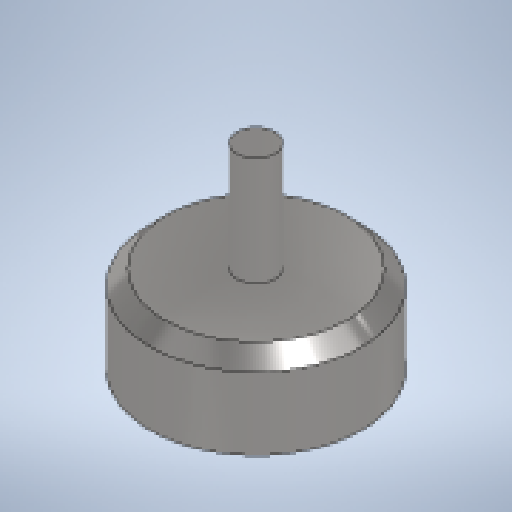
# Autodesk Inventor part: CAN
Saved by Autodesk Inventor 2023.2 (Build 272271000, 271)
## iProperties
Created: 2024-01-31
Part Number: CAN
Material: Stainless Steel
Document SubType Name: Modeling
Designer: Nathan Cai
Density: 8 g/cm^3
Appearance: Smooth - Black
Author: Nathan Cai
Autodesk Inventor part; units mm, degrees
ref_plane "YZ Plane" through (0, 0, 0) normal (1, 0, 0) x (0, 1, 0)
ref_plane "XZ Plane" through (0, 0, 0) normal (0, 1, 0) x (-1, 0, 0)
ref_plane "XY Plane" through (0, 0, 0) normal (0, 0, 1) x (1, 0, 0)
sketch "Sketch1" plane through (0, 0, 0) normal (0, 0, 1) x (1, 0, 0)
  line L0 (0, 0) -> (13.925, 0)
  line L1 (13.925, 0) -> (13.925, -11.5)
  line L2 (13.925, -11.5) -> (0, -11.5) construction
  line L3 (0, -11.5) -> (0, 0) construction
  line L4 (13.925, 0) -> (0, 0)
  line L5 (0, 0) -> (0, -3.5)
  line L6 (0, -3.5) -> (13.925, -3.5)
  line L7 (13.925, -3.5) -> (13.925, 0)
  line L8 (13.925, 0) -> (11.925, 0)
  line L9 (11.925, 0) -> (11.925, -6)
  line L10 (11.925, -6) -> (13.925, -6)
  line L11 (13.925, -6) -> (13.925, 0)
  line L12 (13.925, -6) -> (13.175, -6)
  line L13 (13.175, -6) -> (13.175, -11.5)
  line L14 (13.175, -11.5) -> (13.925, -11.5)
  line L15 (13.925, -11.5) -> (13.925, -6)
  line L16 (0, 0) -> (2.5, 0)
  line L17 (2.5, 0) -> (2.5, 14.25)
  line L18 (2.5, 14.25) -> (0, 14.25)
  line L19 (0, 14.25) -> (0, 0)
  line L20 (0, -3.5) -> (2, -3.5)
  line L21 (2, -3.5) -> (2, -6.5)
  line L22 (2, -6.5) -> (0, -6.5)
  line L23 (0, -6.5) -> (0, -3.5)
  line L24 (2, -6.5) -> (4.5, -3.5)
  line L25 (0, -3.5) -> (1.5, -3.5)
  line L26 (1.5, -3.5) -> (1.5, -6.5)
  line L27 (1.5, -6.5) -> (0, -6.5)
  line L28 (0, -6.5) -> (0, -3.5)
  line L29 (1.5, -6.5) -> (0, -6.5)
  line L30 (0, -6.5) -> (0, -0.5)
  line L31 (0, -0.5) -> (1.5, -0.5)
  line L32 (1.5, -0.5) -> (1.5, -6.5)
  point P0 (11.925, -3.5)
  point P1 (1.5, -3.5)
  point P2 (1.5, -3.5)
  dimension "d0" = 13.925
  dimension "d1" = 11.5
  dimension "d2" = 3.5
  dimension "d3" = 2
  dimension "d5" = 5.5
  dimension "d6" = 0.75
  dimension "d7" = 2.5
  dimension "d8" = 14.25
  dimension "d13" = 2
  dimension "d14" = 3
  dimension "d15" = 4.5
  dimension "d16" = 1.5
  dimension "d53" = 6
  constraints: 66 end point, 16 parallel, 8 horizontal, 8 perpendicular, 5 point on line
  measures "d0" distance of L1.end L2.end
  measures "d1" distance of L0.end L1.end
  measures "d2" distance of L5.end L4.end
  measures "d3" distance of L10.end L9.end
  measures "d5" distance between parallel lines of L2 L10
  measures "d6" distance of L14.end L13.end
  measures "d7" distance of L18.end L17.end
  measures "d8" distance of L17.end L16.end
  measures "d13" distance of L21.end L22.end
  measures "d14" distance of L20.end L21.end
  measures "d15" distance from line of L3 L24.end
  measures "d16" distance of L26.end L27.end
  measures "d53" distance of L29.end L30.end
revolve "Revolution1" add sketch "Sketch1" angle 360 about axis through (0, 14.25, 0) along (0, -1, 0) contours L19 L18 L17 L0 | L0 L9 L6 L32 L31 L5 | L0 L1 L6 L9 | L6 L1 L10 L9 | L6 L21 L22 L26 | L24 L21 L6 | L1 L14 L13 L10
chamfer "Chamfer1" distance 2 angle 45 1 edges at (-13.925, 0, 0)
sketch "Sketch4" plane through (0, -3.5, 0) normal (0, -1, 0) x (1, 0, 0)
  line L0 (0, 0) -> (0, 13.925) construction
  circle A0 centre (0, 0) radius 13.925 projected
  circle A1 centre (0, 0) radius 11.925 projected
  circle A2 centre (0, 0) radius 4.5 projected
  arc A3 (-1.9387, 6.0086) -> (1.9387, 6.0086) centre (0, 6.5) ccw
  line L1 (-1, -13.889) -> (1, -13.889) construction
  line L2 (1, -13.889) -> (1, -4.3875) construction
  line L3 (1, -4.3875) -> (-1, -4.3875) construction
  line L4 (-1, -4.3875) -> (-1, -13.889) construction
  line L5 (-1, -13.889) -> (1, -4.3875) construction
  line L6 (1, -13.889) -> (-1, -4.3875) construction
  circle A4 centre (0, 0) radius 4.5 projected
  circle A5 centre (0, 0) radius 11.925 projected
  line L7 (-3.319, 11.4538) -> (-1.9387, 6.0086)
  line L8 (3.4812, 12.0939) -> (1.9387, 6.0086)
  line L9 (2.0542, -4.0038) -> (8.1617, -11.2824) construction
  line L10 (9.6938, -9.9968) -> (3.5863, -2.7182) construction
  line L11 (4.1472, -1.7467) -> (13.5044, -3.3966) construction
  line L12 (13.8517, -1.427) -> (4.4945, 0.2229) construction
  line L13 (4.2997, 1.3277) -> (12.5283, 6.0785) construction
  line L14 (11.5283, 7.8105) -> (3.2997, 3.0598) construction
  line L15 (2.4403, 3.7809) -> (5.69, 12.7094) construction
  line L16 (3.8106, 13.3935) -> (0.5609, 4.4649) construction
  line L17 (-0.5609, 4.4649) -> (-3.8106, 13.3935) construction
  line L18 (-5.69, 12.7094) -> (-2.4403, 3.7809) construction
  line L19 (-3.2997, 3.0598) -> (-11.5283, 7.8105) construction
  line L20 (-12.5283, 6.0785) -> (-4.2997, 1.3277) construction
  line L21 (-4.4945, 0.2229) -> (-13.8517, -1.427) construction
  line L22 (-13.5044, -3.3966) -> (-4.1472, -1.7467) construction
  line L23 (-3.5863, -2.7182) -> (-9.6938, -9.9968) construction
  line L24 (-8.1617, -11.2824) -> (-2.0542, -4.0038) construction
  line L25 (-5.1071, 11.5022) -> (-2.3771, 5.849)
  arc A6 (-5.3474, 3.3567) -> (-2.3771, 5.849) centre (-4.1781, 4.9793) ccw
  line L26 (-9.9049, 6.6407) -> (-5.3474, 3.3567)
  line L27 (-11.3057, 5.5284) -> (-5.5806, 2.9526)
  arc A7 (-6.2539, -0.8659) -> (-5.5806, 2.9526) centre (-6.4013, 1.1287) ccw
  line L28 (-11.8561, -1.2796) -> (-6.2539, -0.8659)
  line L29 (-12.2143, -3.0321) -> (-6.1729, -1.3253)
  arc A8 (-4.2342, -4.6832) -> (-6.1729, -1.3253) centre (-5.6292, -3.25) ccw
  line L30 (-8.2598, -8.6012) -> (-4.2342, -4.6832)
  line L31 (-7.4077, -10.1739) -> (-3.8768, -4.9831)
  arc A9 (-0.2333, -6.3093) -> (-3.8768, -4.9831) centre (-2.2231, -6.108) ccw
  line L32 (-0.7986, -11.8982) -> (-0.2333, -6.3093)
  line L33 (0.8651, -12.5552) -> (0.2333, -6.3093)
  arc A10 (3.8768, -4.9831) -> (0.2333, -6.3093) centre (2.2231, -6.108) ccw
  line L34 (7.0363, -9.6279) -> (3.8768, -4.9831)
  line L35 (8.733, -9.0618) -> (4.2342, -4.6832)
  arc A11 (6.1729, -1.3253) -> (4.2342, -4.6832) centre (5.6292, -3.25) ccw
  line L36 (11.5788, -2.8526) -> (6.1729, -1.3253)
  line L37 (12.5147, -1.3283) -> (6.2539, -0.8659)
  arc A12 (5.5806, 2.9526) -> (6.2539, -0.8659) centre (6.4013, 1.1287) ccw
  line L38 (10.7035, 5.2575) -> (5.5806, 2.9526)
  line L39 (10.4406, 7.0268) -> (5.3474, 3.3567)
  arc A13 (2.3771, 5.849) -> (5.3474, 3.3567) centre (4.1781, 4.9793) ccw
  line L40 (4.8199, 10.9075) -> (2.3771, 5.849)
  arc A14 (-2.2939, 11.7023) -> (-3.0709, 10.4752) centre (-2.1016, 10.721) ccw
  arc A15 (3.0709, 10.4752) -> (2.2939, 11.7023) centre (2.1016, 10.721) ccw
  arc A16 (-4.3809, 9.9985) -> (-5.7648, 10.439) centre (-5.2814, 9.5636) ccw
  arc A17 (-9.2793, 7.49) -> (-9.0858, 6.0506) centre (-8.5012, 6.8619) ccw
  arc A18 (-9.7828, 4.8433) -> (-11.1262, 4.2912) centre (-10.1932, 3.9313) ccw
  arc A19 (-11.9228, -0.227) -> (-10.8494, -1.2053) centre (-10.923, -0.208) ccw
  arc A20 (-10.6073, -2.5781) -> (-11.2814, -3.8645) centre (-10.3354, -3.5405) ccw
  arc A21 (-8.9875, -7.8378) -> (-7.5364, -7.8971) centre (-8.2338, -7.1805) ccw
  arc A22 (-6.4685, -8.7932) -> (-6.158, -10.212) centre (-5.6416, -9.3556) ccw
  arc A23 (-1.8468, -11.7811) -> (-0.697, -10.8938) centre (-1.6919, -10.7932) ccw
  arc A24 (0.697, -10.8938) -> (1.8468, -11.7811) centre (1.6919, -10.7932) ccw
  arc A25 (6.158, -10.212) -> (6.4685, -8.7932) centre (5.6416, -9.3556) ccw
  arc A26 (7.5364, -7.8971) -> (8.9875, -7.8378) centre (8.2338, -7.1805) ccw
  arc A27 (11.2814, -3.8645) -> (10.6073, -2.5781) centre (10.3354, -3.5405) ccw
  arc A28 (10.8494, -1.2053) -> (11.9228, -0.227) centre (10.923, -0.208) ccw
  arc A29 (11.1262, 4.2912) -> (9.7828, 4.8433) centre (10.1932, 3.9313) ccw
  arc A30 (9.0858, 6.0506) -> (9.2793, 7.49) centre (8.5012, 6.8619) ccw
  arc A31 (5.7648, 10.439) -> (4.3809, 9.9985) centre (5.2814, 9.5636) ccw
  point P0 (0, -9.1383)
  point P1 (-5.69, 12.7094)
  point P2 (-11.5283, 7.8105)
  point P3 (-12.5283, 6.0785)
  point P4 (-13.8517, -1.427)
  point P5 (-13.5044, -3.3966)
  point P6 (-8.1617, -11.2824)
  point P7 (-1, -13.889)
  point P8 (1, -13.889)
  point P9 (8.1617, -11.2824)
  point P10 (9.6938, -9.9968)
  point P11 (13.5044, -3.3966)
  point P12 (13.8517, -1.427)
  point P13 (12.5283, 6.0785)
  point P14 (11.5283, 7.8105)
  point P15 (5.69, 12.7094)
  point P16 (9.0858, 6.0506)
  point P17 (11.1262, 4.2912)
  point P18 (10.8494, -1.2053)
  point P19 (11.9228, -0.227)
  point P20 (10.6073, -2.5781)
  point P21 (8.9875, -7.8378)
  point P22 (6.4685, -8.7932)
  point P23 (0.697, -10.8938)
  point P24 (1.8468, -11.7811)
  point P25 (-1.8468, -11.7811)
  point P26 (-0.697, -10.8938)
  point P27 (-10.6073, -2.5781)
  point P28 (-10.8494, -1.2053)
  point P29 (-9.2793, 7.49)
  point P30 (-9.0858, 6.0506)
  point P31 (-5.7648, 10.439)
  point P32 (2.2939, 11.7023)
  point P33 (-2.2939, 11.7023)
  dimension "d31" = 4
  dimension "d32" = 2
  dimension "d39" = 360
  dimension "d43" = 360
  dimension "d45" = 2
  dimension "d48" = 360
  constraints: 82 end point, 60 point on circle, 27 centre point, 20 point on line, 4 symmetric about line, 4 tangent, 2 midpoint, 2 parallel, 1 horizontal, 1 perpendicular, 1 vertical, 220 other
  measures "d31" diameter of A3
  measures "d32" distance of L3.end L2.end
  measures "d45" diameter of A14
extrude "Extrusion2" cut sketch "Sketch4" against normal blind 3 contours A1 A28 L37 A12 L38 A29 | A30 L39 A13 L40 A31 A1 | A1 A26 L35 A11 L36 A27 | A3 L7 A14 A1 A15 L8 | A10 L34 A25 A1 A24 L33 | A6 L26 A17 A1 A16 L25 | A9 L32 A23 A1 A22 L31 | A7 L28 A19 A1 A18 L27 | A8 L30 A21 A1 A20 L29
sketch "Sketch2" plane through (0, 0, 0) normal (0, 1, 0) x (1, 0, 0)
  circle A0 centre (0, 0) radius 1.5 projected
  circle A1 centre (0, 0) radius 11.5
  line L0 (0, 0) -> (0, 13.925) construction
  circle A2 centre (0, 0) radius 13.925 projected
  line L1 (-1, 16.3936) -> (-1, 11.4564)
  line L2 (-1, 11.4564) -> (1, 11.4564) construction
  line L3 (1, 11.4564) -> (1, 16.3936)
  line L4 (1, 16.3936) -> (-1, 16.3936)
  line L5 (-1, 16.3936) -> (1, 11.4564) construction
  line L6 (-1, 11.4564) -> (1, 16.3936) construction
  line L7 (-11.3036, 11.9154) -> (-8.1301, 8.1334)
  line L8 (-8.1301, 8.1334) -> (-6.598, 9.4189) construction
  line L9 (-6.598, 9.4189) -> (-9.7715, 13.201)
  line L10 (-9.7715, 13.201) -> (-11.3036, 11.9154)
  line L11 (-16.3182, 1.8619) -> (-11.456, 1.0046)
  line L12 (-11.456, 1.0046) -> (-11.1087, 2.9742) construction
  line L13 (-11.1087, 2.9742) -> (-15.9709, 3.8315)
  line L14 (-15.9709, 3.8315) -> (-16.3182, 1.8619)
  line L15 (-13.6972, -9.0628) -> (-9.4216, -6.5942)
  line L16 (-9.4216, -6.5942) -> (-10.4216, -4.8622) construction
  line L17 (-10.4216, -4.8622) -> (-14.6972, -7.3308)
  line L18 (-14.6972, -7.3308) -> (-13.6972, -9.0628)
  line L19 (-4.6672, -15.7469) -> (-2.9786, -11.1076)
  line L20 (-2.9786, -11.1076) -> (-4.858, -10.4235) construction
  line L21 (-4.858, -10.4235) -> (-6.5466, -15.0629)
  line L22 (-6.5466, -15.0629) -> (-4.6672, -15.7469)
  line L23 (6.5466, -15.0629) -> (4.858, -10.4235)
  line L24 (4.858, -10.4235) -> (2.9786, -11.1076) construction
  line L25 (2.9786, -11.1076) -> (4.6672, -15.7469)
  line L26 (4.6672, -15.7469) -> (6.5466, -15.0629)
  line L27 (14.6972, -7.3308) -> (10.4216, -4.8622)
  line L28 (10.4216, -4.8622) -> (9.4216, -6.5942) construction
  line L29 (9.4216, -6.5942) -> (13.6972, -9.0628)
  line L30 (13.6972, -9.0628) -> (14.6972, -7.3308)
  line L31 (15.9709, 3.8315) -> (11.1087, 2.9742)
  line L32 (11.1087, 2.9742) -> (11.456, 1.0046) construction
  line L33 (11.456, 1.0046) -> (16.3182, 1.8619)
  line L34 (16.3182, 1.8619) -> (15.9709, 3.8315)
  line L35 (9.7715, 13.201) -> (6.598, 9.4189)
  line L36 (6.598, 9.4189) -> (8.1301, 8.1334) construction
  line L37 (8.1301, 8.1334) -> (11.3036, 11.9154)
  line L38 (11.3036, 11.9154) -> (9.7715, 13.201)
  arc A3 (6.3519, 11.0119) -> (2.2125, 12.5185) centre (0, 0) ccw construction
  arc A4 (6.9577, 12.0622) -> (2.4235, 13.7125) centre (0, 0) ccw
  arc A5 (5.746, 9.9616) -> (2.0015, 11.3245) centre (0, 0) ccw
  arc A6 (5.746, 9.9616) -> (6.9577, 12.0622) centre (6.3519, 11.0119) ccw
  arc A7 (2.4235, 13.7125) -> (2.0015, 11.3245) centre (2.2125, 12.5185) ccw
  arc A8 (-6.9577, 12.0622) -> (-5.746, 9.9616) centre (-6.3519, 11.0119) ccw
  arc A9 (-2.4235, 13.7125) -> (-6.9577, 12.0622) centre (0, 0) ccw
  arc A10 (-2.2125, 12.5185) -> (-6.3519, 11.0119) centre (0, 0) ccw construction
  arc A11 (-2.0015, 11.3245) -> (-2.4235, 13.7125) centre (-2.2125, 12.5185) ccw
  arc A12 (-2.0015, 11.3245) -> (-5.746, 9.9616) centre (0, 0) ccw
  arc A13 (-13.0833, 4.7679) -> (-10.8049, 3.9375) centre (-11.9441, 4.3527) ccw
  arc A14 (-10.6707, 8.9466) -> (-13.0833, 4.7679) centre (0, 0) ccw
  arc A15 (-9.7416, 8.1675) -> (-11.9441, 4.3527) centre (0, 0) ccw construction
  arc A16 (-8.8125, 7.3885) -> (-10.6707, 8.9466) centre (-9.7416, 8.1675) ccw
  arc A17 (-8.8125, 7.3885) -> (-10.8049, 3.9375) centre (0, 0) ccw
  arc A18 (-13.0871, -4.7574) -> (-10.808, -3.9289) centre (-11.9476, -4.3432) ccw
  arc A19 (-13.925, -0.0056) -> (-13.0871, -4.7574) centre (0, 0) ccw
  arc A20 (-12.7125, -0.0051) -> (-11.9476, -4.3432) centre (0, 0) ccw construction
  arc A21 (-11.5, -0.0046) -> (-13.925, -0.0056) centre (-12.7125, -0.0051) ccw
  arc A22 (-11.5, -0.0046) -> (-10.808, -3.9289) centre (0, 0) ccw
  arc A23 (-6.9673, -12.0566) -> (-5.754, -9.957) centre (-6.3606, -11.0068) ccw
  arc A24 (-10.6636, -8.9551) -> (-6.9673, -12.0566) centre (0, 0) ccw
  arc A25 (-9.7351, -8.1753) -> (-6.3606, -11.0068) centre (0, 0) ccw construction
  arc A26 (-8.8066, -7.3956) -> (-10.6636, -8.9551) centre (-9.7351, -8.1753) ccw
  arc A27 (-8.8066, -7.3956) -> (-5.754, -9.957) centre (0, 0) ccw
  arc A28 (2.4126, -13.7144) -> (1.9924, -11.3261) centre (2.2025, -12.5202) ccw
  arc A29 (-2.4126, -13.7144) -> (2.4126, -13.7144) centre (0, 0) ccw
  arc A30 (-2.2025, -12.5202) -> (2.2025, -12.5202) centre (0, 0) ccw construction
  arc A31 (-1.9924, -11.3261) -> (-2.4126, -13.7144) centre (-2.2025, -12.5202) ccw
  arc A32 (-1.9924, -11.3261) -> (1.9924, -11.3261) centre (0, 0) ccw
  arc A33 (10.6636, -8.9551) -> (8.8066, -7.3956) centre (9.7351, -8.1753) ccw
  arc A34 (6.9673, -12.0566) -> (10.6636, -8.9551) centre (0, 0) ccw
  arc A35 (6.3606, -11.0068) -> (9.7351, -8.1753) centre (0, 0) ccw construction
  arc A36 (5.754, -9.957) -> (6.9673, -12.0566) centre (6.3606, -11.0068) ccw
  arc A37 (5.754, -9.957) -> (8.8066, -7.3956) centre (0, 0) ccw
  arc A38 (13.925, -0.0056) -> (11.5, -0.0046) centre (12.7125, -0.0051) ccw
  arc A39 (13.0871, -4.7574) -> (13.925, -0.0056) centre (0, 0) ccw
  arc A40 (11.9476, -4.3432) -> (12.7125, -0.0051) centre (0, 0) ccw construction
  arc A41 (10.808, -3.9289) -> (13.0871, -4.7574) centre (11.9476, -4.3432) ccw
  arc A42 (10.808, -3.9289) -> (11.5, -0.0046) centre (0, 0) ccw
  arc A43 (10.6707, 8.9466) -> (8.8125, 7.3885) centre (9.7416, 8.1675) ccw
  arc A44 (13.0833, 4.7679) -> (10.6707, 8.9466) centre (0, 0) ccw
  arc A45 (11.9441, 4.3527) -> (9.7416, 8.1675) centre (0, 0) ccw construction
  arc A46 (10.8049, 3.9375) -> (13.0833, 4.7679) centre (11.9441, 4.3527) ccw
  arc A47 (10.8049, 3.9375) -> (8.8125, 7.3885) centre (0, 0) ccw
  point P0 (-8.9508, 10.6672)
  point P1 (-13.7134, 2.4181)
  point P2 (-12.0594, -6.9625)
  point P3 (-4.7626, -13.0852)
  point P4 (4.7626, -13.0852)
  point P5 (12.0594, -6.9625)
  point P6 (13.7134, 2.4181)
  point P7 (8.9508, 10.6672)
  point P8 (-1, 11.4564)
  point P9 (-8.1301, 8.1334)
  point P10 (-11.456, 1.0046)
  point P11 (-9.4216, -6.5942)
  point P12 (-2.9786, -11.1076)
  point P13 (4.858, -10.4235)
  point P14 (10.4216, -4.8622)
  point P15 (11.1087, 2.9742)
  point P16 (-8.1617, 11.2824)
  point P17 (-7.2807, 10.2325)
  point P18 (-5.746, 9.9616)
  point P19 (-2.0015, 11.3245)
  point P20 (-1, 12.5185)
  point P21 (-1, 13.889)
  point P22 (-13.5044, 3.3966)
  point P23 (-12.1547, 3.1586)
  point P24 (-8.8125, 7.3885)
  point P25 (-8.8128, 8.9469)
  point P26 (-9.6938, 9.9968)
  point P27 (-12.5283, -6.0785)
  point P28 (-11.3413, -5.3932)
  point P29 (-10.808, -3.9289)
  point P30 (-11.5, -0.0046)
  point P31 (-12.502, 1.189)
  point P32 (-13.8517, 1.427)
  point P33 (-5.69, -12.7094)
  point P34 (-5.2213, -11.4215)
  point P35 (-5.754, -9.957)
  point P36 (-8.8066, -7.3956)
  point P37 (-10.3413, -7.1253)
  point P38 (-11.5283, -7.8105)
  point P39 (3.8106, -13.3935)
  point P40 (3.3419, -12.1055)
  point P41 (1.9924, -11.3261)
  point P42 (-3.3419, -12.1055)
  point P43 (-3.8106, -13.3935)
  point P44 (11.5283, -7.8105)
  point P45 (10.3413, -7.1253)
  point P46 (5.754, -9.957)
  point P47 (5.2213, -11.4215)
  point P48 (5.69, -12.7094)
  point P49 (13.8517, 1.427)
  point P50 (12.502, 1.189)
  point P51 (11.5, -0.0046)
  point P52 (10.808, -3.9289)
  point P53 (11.3413, -5.3932)
  point P54 (12.5283, -6.0785)
  point P55 (9.6938, 9.9968)
  point P56 (8.8128, 8.9469)
  point P57 (8.8125, 7.3885)
  point P58 (10.8049, 3.9375)
  point P59 (12.1547, 3.1586)
  point P60 (13.5044, 3.3966)
  point P61 (1, 12.5185)
  point P62 (2.0015, 11.3245)
  point P63 (7.2807, 10.2325)
  point P64 (8.1617, 11.2824)
  point P65 (1, 13.889)
  dimension "d17" = 23
  dimension "d18" = 2
  dimension "d21" = 360
  dimension "d25" = 360
  constraints: 90 point on circle, 78 end point, 45 centre point, 6 tangent, 3 parallel, 2 coincident, 2 midpoint, 1 perpendicular, 1 vertical, 216 other
  measures "d18" distance of L2.end L1.end
extrude "Extrusion1" cut sketch "Sketch2" against normal blind 5 contours A38 A2 A41 A1 | L33 A2 A38 | A1 A43 A2 A46 | A46 A2 L31 | A41 A2 L27 | L37 A2 A43 | A33 A2 A36 A1 | L29 A2 A33 | A1 A7 A2 A6 | A6 A2 L35 | A36 A2 L23 | L3 A2 A7 | A28 A2 A31 A1 | L25 A2 A28 | A1 A8 A2 A11 | A11 A2 L1 | A31 A2 L19 | L9 A2 A8 | A23 A2 A26 A1 | L21 A2 A23 | A1 A13 A2 A16 | A16 A2 L7 | A26 A2 L15 | L13 A2 A13 | A18 A2 A21 A1 | L17 A2 A18 | A21 A2 L11
thread "Thread1" size "M5x0.8" class "6g" standard "ANSI Metric M Profile" length 10
sketch "Sketch5" plane through (0, 0, 0) normal (0, 0, 1) x (1, 0, 0)
  line L0 (0, 0) -> (0, -11.5) construction
  line L1 (-13.175, -11.5) -> (13.175, -11.5) projected
  circle A0 centre (0, -2) radius 1.25
  line L2 (1.9924, 0) -> (-1.9924, 0) projected
  point P0 (0, -0.75)
  dimension "d52" = 2.5
  dimension "d55" = 0.75
  constraints: 2 end point, 2 point on line, 1 midpoint, 1 vertical alignment, 2 other
  measures "d55" distance from line of L2 point (0, -0.75)
extrude "Extrusion3" cut sketch "Sketch5" along normal through all
body "Solid1"
